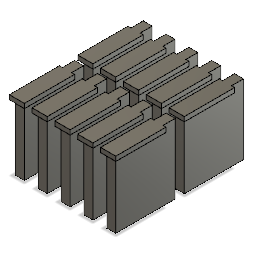
10card v2 (1) (Autodesk Fusion 360 design; units mm, degrees)
Autodesk Fusion 360 part; units mm, degrees
sketch "Sketch1" plane through (0, 0, 0) normal (0, 1, 0) x (1, 0, 0)
  line L0 (0, 0) -> (6, 0)
  line L1 (6, 0) -> (6, 39)
  line L2 (6, 39) -> (0, 39)
  line L3 (0, 39) -> (0, 0)
  dimension "d1" = 6
  dimension "d2" = 39
  constraint horizontal L0
  constraint vertical L1
  constraint horizontal L2
  constraint vertical L3
  constraint coincident L0.start L3.end
  measures "d1" distance of L0.start L0.end
  measures "d2" distance of L0.start L2.end
extrude "Extrude1" add sketch "Sketch1" along normal blind 46 makes body 1
sketch "Sketch2" plane through (6, 0, 0) normal (1, 0, 0) x (0, 0, -1)
  line L0 (0, 0) -> (39, 0)
  line L1 (39, 0) -> (39, 46)
  line L2 (39, 46) -> (0, 46)
  line L3 (0, 46) -> (0, 0)
  line L4 (0, 46) -> (39, 46)
  line L5 (39, 46) -> (39, 43)
  line L6 (39, 43) -> (0, 43)
  line L7 (0, 43) -> (0, 46)
  dimension "d5" = 3
  constraint horizontal L4
  constraint vertical L5
  constraint horizontal L6
  constraint vertical L7
  constraint coincident L2.end L3.start
  measures "d5" distance of L2.end L6.end
extrude "Extrude2" add sketch "Sketch2" along normal blind 3 contours L1 L2 L3 L4 L5 L6 L7 bodies 1
sketch "Sketch3" plane through (0, 0, 0) normal (-1, 0, 0) x (0, 0, 1)
  line L0 (-39, 0) -> (0, 0)
  line L1 (0, 0) -> (0, 46)
  line L2 (0, 46) -> (-39, 46)
  line L3 (-39, 46) -> (-39, 0)
  line L4 (-39, 46) -> (0, 46)
  line L5 (0, 46) -> (0, 43)
  line L6 (0, 43) -> (-39, 43)
  line L7 (-39, 43) -> (-39, 46)
  dimension "d8" = 3
  constraint horizontal L4
  constraint vertical L5
  constraint horizontal L6
  constraint vertical L7
  constraint coincident L2.end L3.start
  measures "d8" distance of L2.end L6.end
extrude "Extrude3" add sketch "Sketch3" along normal blind 3 contours L1 L2 L3 L4 L5 L6 L7 bodies 1
sketch "Sketch4" plane through (0, 0, 0) normal (0, 0, 1) x (1, 0, 0)
  line L0 (0, 0) -> (6, 0)
  line L1 (6, 0) -> (6, 43)
  line L2 (6, 43) -> (9, 43)
  line L3 (9, 43) -> (9, 46)
  line L4 (9, 46) -> (-3, 46)
  line L5 (-3, 46) -> (-3, 43)
  line L6 (-3, 43) -> (0, 43)
  line L7 (0, 43) -> (0, 0)
  line L8 (-3, 46) -> (9, 46)
  line L9 (9, 46) -> (9, 43)
  line L10 (9, 43) -> (-3, 43)
  line L11 (-3, 43) -> (-3, 46)
  constraint horizontal L8
  constraint vertical L9
  constraint horizontal L10
  constraint vertical L11
  constraint coincident L2.end L3.start
  constraint coincident L4.end L5.start
extrude "Extrude4" add sketch "Sketch4" along normal blind 2 contours L2 L3 L4 L5 L6 L8 L9 L10 L11 bodies 1
sketch "Sketch5" plane through (0, 0, -39) normal (0, 0, -1) x (-1, 0, 0)
  line L0 (-6, 0) -> (0, 0)
  line L1 (0, 0) -> (0, 43)
  line L2 (0, 43) -> (3, 43)
  line L3 (3, 43) -> (3, 46)
  line L4 (3, 46) -> (-9, 46)
  line L5 (-9, 46) -> (-9, 43)
  line L6 (-9, 43) -> (-6, 43)
  line L7 (-6, 43) -> (-6, 0)
  line L8 (-9, 46) -> (3, 46)
  line L9 (3, 46) -> (3, 43)
  line L10 (3, 43) -> (-9, 43)
  line L11 (-9, 43) -> (-9, 46)
  constraint horizontal L8
  constraint vertical L9
  constraint horizontal L10
  constraint vertical L11
  constraint coincident L2.end L3.start
  constraint coincident L4.end L5.start
extrude "Extrude5" add sketch "Sketch5" along normal blind 2 contours L2 L3 L4 L5 L6 L8 L9 L10 L11 bodies 1
extrude "Extrude6" cut 1 faces at (5, 45, -41) along direction (0, 0, 1) blind 10 on bodies 1 bodies 1
extrude "Extrude7" cut 1 faces at (-3, 45, -20) along direction (1, 0, 0) blind 1 on bodies 1 bodies 1
extrude "Extrude8" cut 1 faces at (9, 45, -9) along direction (-1, 0, 0) blind 1 on bodies 1 bodies 1
copy_body "CopyPasteBodies5" bodies 1 makes body 2
move_body "Move5" bodies 2 to x (1, 0, 0) y (0, 1, 0) z (0, 0, 1) at (15, 0, 0)
copy_body "CopyPasteBodies6" bodies 1 2 makes body 3 makes body 4
move_body "Move6" bodies 3 4 to x (1, 0, 0) y (0, 1, 0) z (0, 0, 1) at (30, 0, 0)
copy_body "CopyPasteBodies7" bodies 4 makes body 5
move_body "Move7" bodies 5 to x (1, 0, 0) y (0, 1, 0) z (0, 0, 1) at (15, 0, 0)
copy_body "CopyPasteBodies8" bodies 1 5 4 3 2 makes body 6 makes body 7 makes body 8 makes body 9 makes body 10
move_body "Move8" bodies 6 7 8 9 10 to x (1, 0, 0) y (0, 1, 0) z (0, 0, 1) at (0, 0, 45)
extrude "Extrude9" add 10 faces at (62, 43, 8.6667) (47, 43, 8.6667) (32, 43, 8.6667) (17, 43, 8.6667) (2, 43, 11.3333) (2, 43, -36.3333) (17, 43, -36.3333) (32, 43, -36.3333) (47, 43, -36.3333) (62, 43, -36.3333) along direction (0, 1, 0) blind 3 on bodies 1 2 3 4 5 6 7 8 9 10 bodies 7 1 2 3 4 5 6 8 9 10
pasted_body "CopyPasteBodies1" makes body 11
move_body "Move1" [rolled back]
pasted_body "CopyPasteBodies2" makes body 12 makes body 13
move_body "Move2" [rolled back]
pasted_body "CopyPasteBodies3" makes body 14
move_body "Move3" [rolled back]
pasted_body "CopyPasteBodies4" makes body 15 makes body 16 makes body 17 makes body 18 makes body 19
move_body "Move4" [rolled back]
